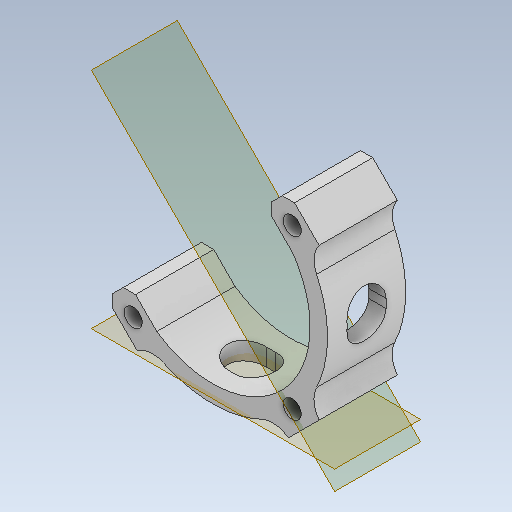
# Autodesk Inventor part: motor_holder_6
Saved by Autodesk Inventor 2020 (Build 240168000, 168)
## iProperties
Created: 2020-03-27
Part Number: motor_holder_6
Material: Generic
Document SubType Name: Modeling
Designer: psrobotics
Density: 1 g/cm^3
Appearance: Default
Author: psrobotics
Autodesk Inventor part; units mm, degrees
ref_plane "YZ Plane" through (0, 0, 0) normal (1, 0, 0) x (0, 1, 0)
sketch "Sketch1" plane through (0, 0, 0) normal (0, 0, 1) x (1, 0, 0)
  line L0 (15.8275, 15.9923) -> (3.9198, 27.9) projected
  arc A0 (-15.9923, -15.8275) -> (15.8275, 15.9923) centre (-0.0824, 0.0824) ccw projected
  line L1 (-15.9923, -15.8275) -> (-27.9, -3.9198) projected
  circle A1 centre (-0.0824, 0.0824) radius 22.5
  circle A2 centre (-0.0824, 0.0824) radius 26.5
  line L2 (-0.0824, 0.0824) -> (18.656, -18.656)
  line L3 (18.656, -18.656) -> (18.3024, -18.3024)
  circle A3 centre (18.3024, -18.3024) radius 3.5
  circle A4 centre (18.3024, 18.3024) radius 3.5
  circle A5 centre (-18.3024, 18.3024) radius 3.5
  circle A6 centre (-18.3024, -18.3024) radius 3.5
  arc A7 (-3.3128, -10.4326) -> (3.1954, -10.418) centre (-0.0824, 0.0824) ccw projected
  line L4 (-13.9943, 30.9649) -> (-40.0339, 57.0045) projected
  arc A8 (-40.0339, 57.0045) -> (-57.0045, 40.0339) centre (-48.5192, 48.5192) ccw projected
  line L5 (-21.7651, 13.2798) -> (-11.5707, 3.0854) projected
  circle A9 centre (18.3024, 18.3024) radius 2.075 projected
  circle A10 centre (-18.3024, -18.3024) radius 2.075 projected
  circle A11 centre (18.3024, -18.3024) radius 2.075 projected
  arc A12 (10.418, -3.1954) -> (10.4326, 3.3128) centre (-0.0824, 0.0824) ccw projected
  line L6 (6.2106, -11.1604) -> (10.4428, -15.3925) projected
  arc A13 (18.148, -21.799) -> (21.799, -18.148) centre (18.3024, -18.3024) ccw projected
  line L7 (15.3925, -10.4428) -> (11.1604, -6.2106) projected
  line L8 (11.1886, 6.3247) -> (15.4397, 10.5377) projected
  arc A14 (21.8005, 18.1879) -> (19.2447, 21.6732) centre (18.3024, 18.3024) ccw projected
  line L9 (10.8169, 15.8116) -> (5.8205, 10.8599) projected
  line L10 (-10.8599, -5.8205) -> (-15.8116, -10.8169) projected
  arc A15 (-21.6732, -19.2447) -> (-18.1879, -21.8005) centre (-18.3024, -18.3024) ccw projected
  line L11 (-10.5377, -15.4397) -> (-6.3247, -11.1886) projected
  arc A16 (23.0573, -12.833) -> (21.799, -18.148) centre (31.7893, -17.7067) ccw projected
  arc A17 (23.0573, -12.833) -> (23.0616, 12.99) centre (-0.0824, 0.0824) ccw projected
  arc A18 (21.8005, 18.1879) -> (23.0616, 12.99) centre (31.7952, 17.8608) ccw projected
  arc A19 (-12.99, -23.0616) -> (-18.1879, -21.8005) centre (-17.8608, -31.7952) ccw projected
  arc A20 (-12.99, -23.0616) -> (12.833, -23.0573) centre (-0.0824, 0.0824) ccw projected
  arc A21 (18.148, -21.799) -> (12.833, -23.0573) centre (17.7067, -31.7893) ccw projected
  arc A22 (-9.6876, -20.2644) -> (9.6143, -20.2209) centre (-0.0824, 0.0824) ccw projected
  arc A23 (-10.5377, -15.4397) -> (-9.6876, -20.2644) centre (-8.4069, -17.5515) ccw projected
  arc A24 (-3.3128, -10.4326) -> (-6.3247, -11.1886) centre (-4.1938, -13.3003) ccw projected
  arc A25 (6.2106, -11.1604) -> (3.1954, -10.418) centre (4.0893, -13.2817) ccw projected
  arc A26 (9.6143, -20.2209) -> (10.4428, -15.3925) centre (8.3215, -17.5138) ccw projected
  arc A27 (20.2209, -9.6143) -> (20.2644, 9.6876) centre (-0.0824, 0.0824) ccw projected
  arc A28 (15.3925, -10.4428) -> (20.2209, -9.6143) centre (17.5138, -8.3215) ccw projected
  arc A29 (10.418, -3.1954) -> (11.1604, -6.2106) centre (13.2817, -4.0893) ccw projected
  arc A30 (11.1886, 6.3247) -> (10.4326, 3.3128) centre (13.3003, 4.1938) ccw projected
  arc A31 (20.2644, 9.6876) -> (15.4397, 10.5377) centre (17.5515, 8.4069) ccw projected
  line L12 (-19.1583, -9.9475) -> (-25.1055, 11.3271) projected
  line L13 (-30.9649, 13.9943) -> (-21.6732, -19.2447) projected
  line L14 (19.2447, 21.6732) -> (-13.9943, 30.9649) projected
  line L15 (-57.0045, 40.0339) -> (-30.9649, 13.9943) projected
  line L16 (-11.3271, 25.1055) -> (9.9475, 19.1583) projected
  circle A32 centre (-48.5192, 48.5192) radius 8.075 projected
  circle A33 centre (-0.0824, 0.0824) radius 6.575 projected
  arc A34 (3.7211, 10.4039) -> (5.8205, 10.8599) centre (4.4127, 12.2805) ccw projected
  arc A35 (3.7211, 10.4039) -> (-1.4268, 10.9999) centre (-0.0824, 0.0824) ccw projected
  arc A36 (-3.0854, 11.5707) -> (-1.4268, 10.9999) centre (-1.6712, 12.9849) ccw projected
  line L17 (-3.0854, 11.5707) -> (-13.2798, 21.7651) projected
  arc A37 (-11.3271, 25.1055) -> (-13.2798, 21.7651) centre (-11.8656, 23.1793) ccw projected
  arc A38 (10.8169, 15.8116) -> (9.9475, 19.1583) centre (9.4091, 17.2321) ccw projected
  arc A39 (-19.1583, -9.9475) -> (-15.8116, -10.8169) centre (-17.2321, -9.4091) ccw projected
  arc A40 (-21.7651, 13.2798) -> (-25.1055, 11.3271) centre (-23.1793, 11.8656) ccw projected
  arc A41 (-10.9999, 1.4268) -> (-11.5707, 3.0854) centre (-12.9849, 1.6712) ccw projected
  arc A42 (-10.9999, 1.4268) -> (-10.4039, -3.7211) centre (-0.0824, 0.0824) ccw projected
  arc A43 (-10.8599, -5.8205) -> (-10.4039, -3.7211) centre (-12.2805, -4.4127) ccw projected
  point P0 (0, 0)
  point P1 (-25.8918, -5.9281)
  point P2 (-21.0455, -16.1286)
  point P3 (-16.104, -21.0258)
  point P4 (16.0253, -20.9603)
  point P5 (20.9603, -16.0253)
  point P6 (21.0258, 16.104)
  point P7 (16.1286, 21.0455)
  point P8 (5.9281, 25.8918)
  point P9 (-0.0824, 0.0824)
  point P10 (15.8275, -20.7773)
  point P11 (20.7773, -15.8275)
  point P12 (20.7661, 15.8164)
  point P13 (15.8387, 20.7884)
  point P14 (-20.7884, -15.8387)
  point P15 (-15.8164, -20.7661)
  point P16 (18.3024, 18.3024)
  point P17 (-18.3024, -18.3024)
  point P18 (-48.5192, 48.5192)
  dimension "d0" = 45
  dimension "d1" = 4
  dimension "d2" = 0.5
  dimension "d3" = 7
  dimension "d6" = 360
  constraints: 6 centre point, 4 end point, 3 coincident, 1 parallel, 1 point on circle, 1 point on line, 9 other
  measures "d0" diameter of A1
  measures "d1" radial gap between concentric circles of A1 A2
  measures "d2" distance of L2.end L3.end
  measures "d3" diameter of A3
ref_plane "Work Plane1" through (-23.6676, -23.5029, 19) normal (0, 0, 1) x (0.9657567, 0.2594493, 0)
extrude "Extrusion1" add sketch "Sketch1" along normal up to surface (19 mm away) contours L0 A4 A2 A9 A0 | L0 L14 A2 A4 | A4 A2 A3 A0 | L0 A2 L14 | A4 A2 A9 | A9 A2 | A2 A9 | A3 A2 A6 A0 | A3 A2 A11 L2 | L2 A11 A2 A3 | A11 A2 L2 | L2 A2 A11 | A3 A2 A11 | A11 A2 | A6 A2 A10 L1 A0 | L1 L13 A2 | L1 A6 A2 L13 | A6 A2 A10 | A10 A2 | A2 A10 picked at (9.4762, 24.5169) picked at (-24.5169, -9.4762)
sketch "Sketch2" plane through (-0.0824, 0.0824, 19) normal (0, 0, 1) x (0.7071068, 0.7071068, 0)
  arc A0 (3.4896, -26.2692) -> (26.2548, -3.5967) centre (0, 0) ccw projected
  arc A1 (26.2548, -3.5967) -> (26.2861, 3.3603) centre (25.8835, -0.1165) ccw projected
  arc A2 (26.2861, 3.3603) -> (22.5, 14) centre (0, 0) ccw projected
  line L0 (22.5, 0) -> (22.5, 14) projected
  arc A3 (-22.5, 0) -> (22.5, 0) centre (0, 0) ccw projected
  line L1 (-22.5, 14) -> (-22.5, 0) projected
  arc A4 (-22.5, 14) -> (-26.2861, 3.3603) centre (0, 0) ccw projected
  arc A5 (-26.2861, 3.3603) -> (-26.2548, -3.5967) centre (-25.8835, -0.1165) ccw projected
  arc A6 (-26.2548, -3.5967) -> (-3.4896, -26.2692) centre (0, 0) ccw projected
  arc A7 (-3.4896, -26.2692) -> (3.4896, -26.2692) centre (0, -26) ccw projected
  line L2 (22.5, 0) -> (22.5, 14) projected
  line L3 (22.5, 0) -> (29.3816, 0)
  line L4 (29.3816, 0) -> (29.3816, 14)
  line L5 (29.3816, 14) -> (22.5, 14)
  line L6 (22.5, 14) -> (22.5, 0)
  arc A8 (-22.5, 0) -> (22.5, 0) centre (0, 0) ccw projected
  line L7 (-22.5, 0) -> (-29.3816, 0)
  line L8 (-29.3816, 0) -> (-29.3816, 14)
  line L9 (-29.3816, 14) -> (-22.5, 14)
  line L10 (-22.5, 14) -> (-22.5, 0)
  arc A9 (-26.2861, 3.3603) -> (-26.2548, -3.5967) centre (-25.8835, -0.1165) ccw projected
  point P0 (0, -0.1165)
  point P1 (-29.3835, -0.1322)
  constraints: 16 end point, 4 parallel, 4 point on circle, 2 horizontal, 2 perpendicular, 2 point on line
ref_plane "Work Plane2" through (-82.9336, -82.5377, 0) normal (0, 0, 1) x (1, 0, 0)
extrude "Extrusion2" add sketch "Sketch2" against normal up to surface (19 mm away) contours A1 A2 L5 L4 | L8 L9 A4 A5
thicken "Thicken1" operation add thickness 10 both sides no extend neighbours yes toward (0.7071068, -0.7071068, 0) faces at (9.1721, 29.1358, 6.3333)
thicken "Thicken2" operation add thickness 10 both sides no extend neighbours yes toward (0.7071068, -0.7071068, 0) faces at (-29.1358, -9.1721, 12.6667)
sketch "Sketch3" plane through (-0.0824, 0.0824, 19) normal (0, 0, 1) x (0.7071068, 0.7071068, 0)
  arc A0 (3.4896, -26.2692) -> (26.2548, -3.5967) centre (0, 0) ccw projected
  arc A1 (26.2548, -3.5967) -> (29.3816, 0) centre (25.8835, -0.1165) ccw projected
  line L0 (29.3816, 0) -> (29.3816, 4) projected
  line L1 (29.3816, 4) -> (22.5, 4) projected
  line L2 (22.5, 0) -> (22.5, 4) projected
  arc A2 (-22.5, 0) -> (22.5, 0) centre (0, 0) ccw projected
  line L3 (-22.5, 4) -> (-22.5, 0) projected
  line L4 (-22.5, 4) -> (-29.3816, 4) projected
  line L5 (-29.3816, 4) -> (-29.3816, 0) projected
  arc A3 (-29.3816, 0) -> (-26.2548, -3.5967) centre (-25.8835, -0.1165) ccw projected
  arc A4 (-26.2548, -3.5967) -> (-3.4896, -26.2692) centre (0, 0) ccw projected
  arc A5 (-3.4896, -26.2692) -> (3.4896, -26.2692) centre (0, -26) ccw projected
  point P0 (0, -0.1165)
hole "Hole1" at (18.3024, 18.3024, 19) at (18.3024, -18.3024, 19) at (-18.3024, -18.3024, 19) direction (0, 0, -1) diameter 4.15 depth 7
sketch "Sketch4" plane through (0, 0, 0) normal (0, 0, -1) x (-1, 0, 0)
  line L0 (23.6867, -17.8651) -> (18.8207, -12.9991) projected
  line L1 (15.9923, -15.8275) -> (18.8207, -12.9991) projected
  arc A0 (-15.8275, 15.9923) -> (15.9923, -15.8275) centre (0.0824, 0.0824) ccw projected
  line L2 (-12.9991, 18.8207) -> (-15.8275, 15.9923) projected
  line L3 (-12.9991, 18.8207) -> (-17.8651, 23.6867) projected
  line L4 (-17.8651, 23.6867) -> (-20.6936, 20.8583) projected
  arc A1 (-20.6936, 20.8583) -> (-21.0258, 16.104) centre (-18.3024, 18.3024) ccw projected
  arc A2 (-16.0253, -20.9603) -> (16.104, -21.0258) centre (0.0824, 0.0824) ccw projected
  arc A3 (-20.9603, -16.0253) -> (-16.0253, -20.9603) centre (-18.3024, -18.3024) ccw projected
  arc A4 (-21.0258, 16.104) -> (-20.9603, -16.0253) centre (0.0824, 0.0824) ccw projected
  arc A5 (16.104, -21.0258) -> (20.8583, -20.6936) centre (18.3024, -18.3024) ccw projected
  line L5 (20.8583, -20.6936) -> (23.6867, -17.8651) projected
  circle A6 centre (-18.3024, 18.3024) radius 2.075 projected
  circle A7 centre (-18.3024, -18.3024) radius 2.075 projected
  circle A8 centre (18.3024, -18.3024) radius 2.075 projected
  point P0 (0, 0)
hole "Hole2" at (18.3024, 18.3024, 0) at (18.3024, -18.3024, 0) at (-18.3024, -18.3024, 0) direction (0, 0, 1) diameter 4.15 depth 7
sketch "Sketch8" plane through (0, 0, 0) normal (0, 0, -1) x (-1, 0, 0)
  circle A0 centre (-18.3024, -18.3024) radius 2.075 projected
  circle A1 centre (-18.3024, 18.3024) radius 2.075 projected
  circle A2 centre (18.3024, -18.3024) radius 2.075 projected
  arc A3 (-20.6936, 20.8583) -> (-21.0258, 16.104) centre (-18.3024, 18.3024) ccw projected
  arc A4 (-21.0258, 16.104) -> (-20.9603, -16.0253) centre (0.0824, 0.0824) ccw projected
  arc A5 (-20.9603, -16.0253) -> (-16.0253, -20.9603) centre (-18.3024, -18.3024) ccw projected
  arc A6 (-16.0253, -20.9603) -> (16.104, -21.0258) centre (0.0824, 0.0824) ccw projected
  arc A7 (16.104, -21.0258) -> (20.8583, -20.6936) centre (18.3024, -18.3024) ccw projected
  line L0 (20.8583, -20.6936) -> (23.6867, -17.8651) projected
  line L1 (23.6867, -17.8651) -> (18.8207, -12.9991) projected
  line L2 (15.9923, -15.8275) -> (18.8207, -12.9991) projected
  arc A8 (-15.8275, 15.9923) -> (15.9923, -15.8275) centre (0.0824, 0.0824) ccw projected
  line L3 (-12.9991, 18.8207) -> (-15.8275, 15.9923) projected
  line L4 (-12.9991, 18.8207) -> (-17.8651, 23.6867) projected
  line L5 (-17.8651, 23.6867) -> (-20.6936, 20.8583) projected
  line L6 (24.4896, -17.4185) -> (19.1863, -12.1152)
  line L7 (19.1863, -12.1152) -> (12.1152, -19.1863)
  line L8 (12.1152, -19.1863) -> (17.4185, -24.4896)
  line L9 (17.4185, -24.4896) -> (24.4896, -17.4185)
  line L10 (24.4896, -17.4185) -> (12.1152, -19.1863) construction
  line L11 (19.1863, -12.1152) -> (17.4185, -24.4896) construction
  line L12 (23.6867, -17.8651) -> (18.8207, -12.9991) projected
  point P0 (0, 0)
  dimension "d49" = 7.5
  dimension "d50" = 10
  constraints: 12 end point, 3 parallel, 2 midpoint, 1 perpendicular
  measures "d49" distance of L6.start L6.end
  measures "d50" distance of L7.end L6.end
extrude "Extrusion5" add sketch "Sketch8" against normal up to surface (19 mm away) contours L8 L7 A8 L2 L1 L0 A7 A6 | A6 A7 L0 L1 L2 A8 L7 L6 L9 L8
sketch "Sketch9" plane through (0, 0, 0) normal (0, 0, -1) x (-1, 0, 0)
  circle A0 centre (18.3024, -18.3024) radius 2.075 projected
  line L0 (14.8502, -21.9213) -> (17.4185, -24.4896) projected
  line L1 (17.4185, -24.4896) -> (24.4896, -17.4185) projected
  line L2 (24.4896, -17.4185) -> (19.1863, -12.1152) projected
  line L3 (19.1863, -12.1152) -> (12.8733, -18.4282) projected
  arc A1 (-15.8275, 15.9923) -> (12.8733, -18.4282) centre (0.0824, 0.0824) ccw projected
  line L4 (-12.9991, 18.8207) -> (-15.8275, 15.9923) projected
  line L5 (-12.9991, 18.8207) -> (-17.8651, 23.6867) projected
  line L6 (-17.8651, 23.6867) -> (-20.6936, 20.8583) projected
  arc A2 (-20.6936, 20.8583) -> (-21.0258, 16.104) centre (-18.3024, 18.3024) ccw projected
  arc A3 (-21.0258, 16.104) -> (-20.9603, -16.0253) centre (0.0824, 0.0824) ccw projected
  arc A4 (-20.9603, -16.0253) -> (-16.0253, -20.9603) centre (-18.3024, -18.3024) ccw projected
  arc A5 (-16.0253, -20.9603) -> (14.8502, -21.9213) centre (0.0824, 0.0824) ccw projected
  circle A6 centre (-18.3024, 18.3024) radius 2.075 projected
  circle A7 centre (-18.3024, -18.3024) radius 2.075 projected
  line L7 (-12.1152, 19.1863) -> (-17.4185, 24.4896)
  line L8 (-17.4185, 24.4896) -> (-24.4896, 17.4185)
  line L9 (-24.4896, 17.4185) -> (-19.1863, 12.1152)
  line L10 (-19.1863, 12.1152) -> (-12.1152, 19.1863)
  line L11 (-12.1152, 19.1863) -> (-24.4896, 17.4185) construction
  line L12 (-17.4185, 24.4896) -> (-19.1863, 12.1152) construction
  point P0 (0, 0)
  dimension "d53" = 7.5
  dimension "d54" = 10
  constraints: 12 end point, 3 parallel, 2 midpoint, 1 perpendicular
  measures "d53" distance of L7.start L7.end
  measures "d54" distance of L8.end L7.end
extrude "Extrusion6" add sketch "Sketch9" against normal up to surface (19 mm away) contours L9 L8 L7 L10 A1 L4 L5 L6 A2 A3 | A3 A2 L6 L5 L4 A1 L10 L9
sketch "Sketch10" plane through (0, 0, 0) normal (0, 0, -1) x (-1, 0, 0)
  arc A0 (-21.9213, 14.8502) -> (-20.9603, -16.0253) centre (0.0824, 0.0824) ccw projected
  arc A1 (-20.9603, -16.0253) -> (-16.0253, -20.9603) centre (-18.3024, -18.3024) ccw projected
  arc A2 (-16.0253, -20.9603) -> (14.8502, -21.9213) centre (0.0824, 0.0824) ccw projected
  line L0 (14.8502, -21.9213) -> (17.4185, -24.4896) projected
  line L1 (17.4185, -24.4896) -> (24.4896, -17.4185) projected
  line L2 (24.4896, -17.4185) -> (19.1863, -12.1152) projected
  line L3 (19.1863, -12.1152) -> (12.8733, -18.4282) projected
  arc A3 (-18.4282, 12.8733) -> (12.8733, -18.4282) centre (0.0824, 0.0824) ccw projected
  line L4 (-18.4282, 12.8733) -> (-12.1152, 19.1863) projected
  line L5 (-12.1152, 19.1863) -> (-17.4185, 24.4896) projected
  line L6 (-17.4185, 24.4896) -> (-24.4896, 17.4185) projected
  line L7 (-24.4896, 17.4185) -> (-21.9213, 14.8502) projected
  circle A4 centre (-18.3024, 18.3024) radius 2.075 projected
  circle A5 centre (18.3024, -18.3024) radius 2.075 projected
  circle A6 centre (-18.3024, -18.3024) radius 2.075 projected
  line L8 (-12.1152, -19.1863) -> (-19.1863, -12.1152)
  line L9 (-19.1863, -12.1152) -> (-24.4896, -17.4185)
  line L10 (-24.4896, -17.4185) -> (-17.4185, -24.4896)
  line L11 (-17.4185, -24.4896) -> (-12.1152, -19.1863)
  line L12 (-12.1152, -19.1863) -> (-24.4896, -17.4185) construction
  line L13 (-19.1863, -12.1152) -> (-17.4185, -24.4896) construction
  circle A7 centre (-18.3024, 18.3024) radius 2.075 projected
  line L14 (18.3024, -18.3024) -> (-18.3024, 18.3024)
  line L15 (-18.3024, -18.3024) -> (0.0824, 0.0824)
  point P0 (0, 0)
  point P1 (-14.7839, -21.8549)
  point P2 (-21.8549, -14.7839)
  dimension "d57" = 10
  dimension "d58" = 7.5
  constraints: 16 end point, 2 midpoint, 2 parallel, 2 perpendicular
  measures "d57" distance of L8.start L8.end
  measures "d58" distance of L9.end L8.end
extrude "Extrusion7" add sketch "Sketch10" against normal up to surface (19 mm away) contours A0 A1 A2 L11 L10 L9
fillet "Fillet3" radius 6 4 edges at (14.7839, -21.8549, 9.5) (-14.8502, -21.9213, 9.5) (21.8549, -14.7839, 9.5) (21.9213, 14.8502, 9.5)
thicken "Thicken3" operation add thickness 1 both sides no extend neighbours yes toward (0, 0, 1) faces at (23.5222, 8.4821, 0)
ref_plane "Work Plane6" through (-17.4185, -24.4896, 0) normal (0, 1, 0) x (0, 0, 1)
ref_plane "Work Plane7" through (-3.5355, 3.5355, 1) normal (-0.7071068, -0.7071068, 0) x (0, 0, 1)
sketch "Sketch11" plane through (-17.4185, -24.4896, 0) normal (0, 1, 0) x (0, 0, 1)
  line L0 (1, 6.0801) -> (19, 6.0801) projected
  line L1 (1, 6.0801) -> (1, 28.6742) projected
  line L2 (19, 28.6742) -> (1, 28.6742) projected
  line L3 (19, 28.6742) -> (19, 6.0801) projected
  line L4 (19, 28.6742) -> (19, 6.0801) projected
  line L5 (19, 6.0801) -> (1, 28.6742)
  line L6 (19, 28.6742) -> (1, 28.6742) projected
  line L7 (19, 28.6742) -> (1, 6.0801)
  line L8 (10, 16.3772) -> (10, 18.3772) construction
  line L9 (14.5, 16.3772) -> (14.5, 18.3772)
  line L10 (5.5, 18.3772) -> (5.5, 16.3772)
  arc A0 (5.5, 16.3772) -> (14.5, 16.3772) centre (10, 16.3772) ccw
  arc A1 (14.5, 18.3772) -> (5.5, 18.3772) centre (10, 18.3772) ccw
  point P0 (0, 17.4185)
  point P1 (10, 17.3772)
  dimension "d64" = 1
  dimension "d65" = 9
  constraints: 12 end point, 4 point on circle, 4 tangent, 2 centre point, 2 midpoint, 1 parallel, 1 vertical
  measures "d64" distance of point (10, 17.377) L8.end
  measures "d65" diameter of A1
extrude "Extrusion8" cut sketch "Sketch11" against normal mid plane 10 contours A0 L10 A1 L5 L7 | L7 L5 A0 | L5 L7 A1 L9 A0 | A1 L7 L5
mirror "Mirror3" about plane through (-3.5355, 3.5355, 1) normal (-0.7071068, -0.7071068, 0) of "Extrusion8"
chamfer "Chamfer2" distance 2 angle 45 4 edges at (-19.1863, -12.1152, 10) (-24.4896, -17.4185, 10) (17.4185, 24.4896, 10) (12.1152, 19.1863, 10)
body "Solid1"
